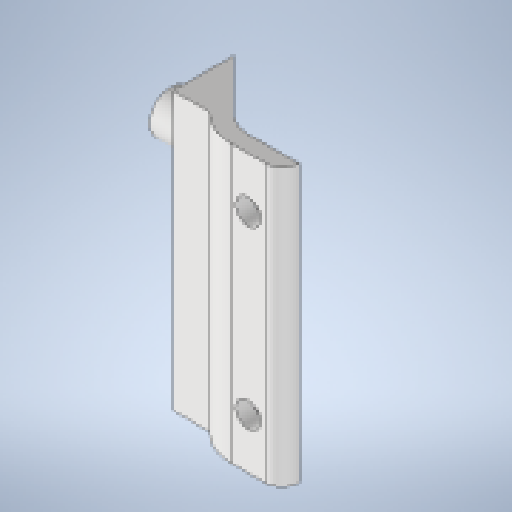
# Autodesk Inventor part: GripperHandleLeft
Saved by Autodesk Inventor 2025.1 (Build 291241000, 241)
## iProperties
Created: 2026-05-06
Part Number: GripperHandleLeft
Material: Generic
Document SubType Name: Modeling
Designer: User
Density: 1 g/cm^3
Appearance: Default
Author: User
## iProperties of the stored document GripperHandleLeft_3DPrint.ipt
Created: 2026-05-06
Part Number: GripperHandleLeft_3DPrint
Material: Generic
Document SubType Name: Modeling
Designer: User
Density: 1 g/cm^3
Appearance: Default
Author: User
Autodesk Inventor part; units mm, degrees
ref_plane "YZ Plane" through (0, 0, 0) normal (1, 0, 0) x (0, 1, 0)
ref_plane "XZ Plane" through (0, 0, 0) normal (0, 1, 0) x (-1, 0, 0)
ref_plane "XY Plane" through (0, 0, 0) normal (0, 0, 1) x (1, 0, 0)
sketch "Sketch1" plane through (0, 0, 0) normal (0, 0, 1) x (1, 0, 0)
  line L0 (122.2883, -16.0055) -> (122.2883, 46.9321) projected
  line L1 (122.2883, -16.0055) -> (128.4096, -16.0055) projected
  line L2 (128.4096, -16.0055) -> (128.4096, 44.4321) projected
  line L3 (136.1877, 44.4321) -> (128.4096, 44.4321) projected
  line L4 (136.1877, 46.9321) -> (136.1877, 44.4321) projected
  line L5 (122.2883, 46.9321) -> (136.1877, 46.9321) projected
  line L6 (3.0607, 16.0055) -> (-1.0607, 16.0055) projected
  line L7 (122.2883, 16.0055) -> (128.4096, 16.0055)
  point P0 (0, 0)
  constraints: 2 end point, 2 point on line
extrude "Extrusion1" add sketch "Sketch1" against normal blind 2 contours L0 L7 L2 L1
sketch "Sketch2" plane through (122.2883, -16.0055, 0) normal (0, -1, 0) x (1, 0, 0)
  line L0 (0, 0) -> (6.1213, 0) projected
  line L1 (0, 0) -> (0, -2) projected
  line L2 (6.1213, -2) -> (0, -2) projected
  line L3 (6.1213, 0) -> (6.1213, -2) projected
  point P0 (-122.2883, 0)
ref_plane "Work Plane1" through (-3.0607, -16.2055, -14.9496) normal (0, 1, 0) x (0.7071068, 0, 0.7071068)
extrude "Extrusion2" add sketch "Sketch2" along normal up to surface (0.2 mm away)
ref_plane "Work Plane2" through (-3.4749, -17.2055, -14.9496) normal (0, -1, 0) x (0.7071068, 0, -0.7071068)
sketch "Sketch3" plane through (122.2883, -16.2055, -2) normal (0, -1, 0) x (1, 0, 0)
  line L0 (0, 2) -> (0, 0)
  line L1 (0, 0) -> (6.1213, 0)
  line L2 (6.1213, 0) -> (6.1213, 2)
  line L3 (6.1213, 2) -> (0, 2)
  arc A0 (-123.3489, 2) -> (-125.3489, 0) centre (-123.3489, 0) ccw
  line L4 (-125.3489, 0) -> (-122.3489, -3)
  line L5 (-122.3489, -3) -> (-118.1063, -3)
  line L6 (-118.1063, -3) -> (-110.278, -10.8283)
  line L7 (-110.278, -10.8283) -> (-110.278, 0)
  line L8 (-110.278, 0) -> (-114.7423, 0)
  line L9 (-114.7423, 0) -> (-114.9849, 0.2426)
  arc A1 (-114.9849, 0.2426) -> (-119.2276, 2) centre (-119.2276, -4) ccw
  line L10 (-119.2276, 2) -> (-123.3489, 2)
  line L11 (-110.278, -10.8283) -> (8.4603, -10.8283)
  line L12 (-110.278, -10.8283) -> (8.4603, -10.8283) construction
  arc A2 (0, 0) -> (-2.8284, -1.1716) centre (0, -4) ccw
  line L13 (-54.1499, -52.493) -> (-2.8284, -1.1716)
  line L14 (-12.4852, -10.8283) -> (-1.6569, -10.8283) construction
  arc A3 (0, 2) -> (-4.2426, 0.2426) centre (0, -4) ccw
  line L15 (-1.1213, -3) -> (-18.8648, -20.7435)
  line L16 (3.1213, -3) -> (-1.1213, -3)
  line L17 (6.1213, 0) -> (3.1213, -3)
  line L18 (-8.9496, -10.8283) -> (81.0504, -10.8283) construction
  line L19 (-8.9496, -10.8283) -> (-8.9496, 0)
  line L20 (-8.9496, -10.8283) -> (1.8787, -10.8283) construction
  line L21 (-8.9496, 0) -> (-4.4853, 0)
  line L22 (-55.5641, -51.0788) -> (-8.9496, -4.4643)
  line L23 (-4.4853, 0) -> (-4.2426, 0.2426)
  point P0 (-122.2883, 2)
extrude "Extrusion3" add sketch "Sketch3" along normal up to surface (1 mm away) contours L3 L2 L1 L0 | L0 A2 L13 L19 L21 L23 A3 | L1 L17 L16 L15 L19 L13 A2
sketch "Sketch4" plane through (122.2883, -16.2055, -2) normal (0, 1, 0) x (1, 0, 0)
  line L0 (-2.8284, 1.1716) -> (-33.605, 31.9482) projected
  arc A0 (-2.8284, 1.1716) -> (0, 0) centre (0, 4) ccw projected
  line L1 (0, -2) -> (0, 0) projected
  arc A1 (-4.2426, -0.2426) -> (0, -2) centre (0, 4) ccw projected
  line L2 (-4.2426, -0.2426) -> (-4.4853, 0) projected
  line L3 (-4.4853, 0) -> (-8.9496, 0) projected
  line L4 (-8.9496, 0) -> (-8.9496, 10.8283) projected
  point P0 (-122.2883, -2)
  point P1 (-8.9496, 7.2928)
extrude "Extrusion4" add sketch "Sketch4" along normal up to surface (32.211 mm away)
fillet "Fillet1" radius 2 1 edges at (128.4096, -0.6, 0)
sketch "Sketch6" plane through (113.3386, -17.2055, -2) normal (-1, 0, 0) x (0, 0, 1)
  circle A0 centre (6.5566, 27.211) radius 35
  line L0 (-7.2928, 1) -> (-7.2928, 33.211) projected
  line L1 (-10.8283, 0) -> (0, 0) projected
  line L2 (0, 33.211) -> (0, 0) projected
  line L3 (0, 33.211) -> (-7.2928, 33.211) projected
  line L4 (-7.2928, 1) -> (-7.2928, 33.211) projected
  line L5 (-7.2928, 1) -> (-10.8283, 1) projected
  line L6 (-10.8283, 1) -> (-10.8283, 0) projected
  line L7 (0, 27.211) -> (-7.2928, 27.211)
  circle A1 centre (-3.6464, 27.211) radius 2.5
  point P0 (2, 17.2055)
  dimension "d16" = 5
  constraints: 2 centre point, 2 end point, 2 point on line, 1 midpoint, 2 other
  measures "d16" diameter of A1
extrude "Extrusion5" add sketch "Sketch6" along normal blind 4 contours A1 L7 | L7 A1
chamfer "Chamfer1" distance 0.5 angle 45 1 edges at (113.3386, 10.0055, -8.1464)
sketch "Sketch7" plane through (109.3386, 10.0055, -5.6464) normal (-1, 0, 0) x (0, 0, 1)
  circle A0 centre (0, 0) radius 2.5 projected
  circle A1 centre (0, 0) radius 1.5
  point P0 (5.6464, -10.0055)
  dimension "d22" = 3
  constraints: 1 centre point, 1 coincident
  measures "d22" diameter of A1
extrude "Extrusion6" cut sketch "Sketch7" against normal through all contours A1
sketch "Sketch8" plane through (0, 0, 0) normal (0, 0, 1) x (1, 0, 0)
  line L0 (126.4096, 16.0055) -> (126.4096, -17.2055) projected
  line L1 (126.4096, 16.0055) -> (122.2883, 16.0055) projected
  line L2 (122.2883, 16.0055) -> (122.2883, -17.2055) projected
  line L3 (122.2883, -17.2055) -> (126.4096, -17.2055) projected
  line L4 (122.2883, 16.0055) -> (119.4598, 16.0055) projected
  line L5 (122.2883, 16.0055) -> (126.4096, 16.0055)
  line L6 (126.4096, 16.0055) -> (126.4096, 12.0055)
  line L7 (126.4096, 12.0055) -> (122.2883, 12.0055)
  line L8 (122.2883, 12.0055) -> (122.2883, 16.0055)
  line L9 (122.2883, -17.2055) -> (126.4096, -17.2055)
  line L10 (126.4096, -17.2055) -> (126.4096, -13.2055)
  line L11 (126.4096, -13.2055) -> (122.2883, -13.2055)
  line L12 (122.2883, -13.2055) -> (122.2883, -17.2055)
  circle A0 centre (124.3489, 9.9448) radius 2.0607
  circle A1 centre (124.3489, -11.1448) radius 2.0607
  circle A2 centre (124.3489, 9.9448) radius 1.5
  circle A3 centre (124.3489, -11.1448) radius 1.5
  point P0 (0, 0)
  dimension "d25" = 4
  dimension "d26" = 4
  dimension "d27" = 3
  dimension "d28" = 3
  constraints: 16 end point, 6 tangent, 4 centre point, 4 parallel, 2 coincident, 2 horizontal, 2 perpendicular, 2 point on line
  measures "d25" distance of L5.end L6.end
  measures "d26" distance of L10.end L9.end
  measures "d27" diameter of A2
  measures "d28" diameter of A3
extrude "Extrusion7" cut sketch "Sketch8" against normal blind 10 contours A2 | A3
body "Solid1"
